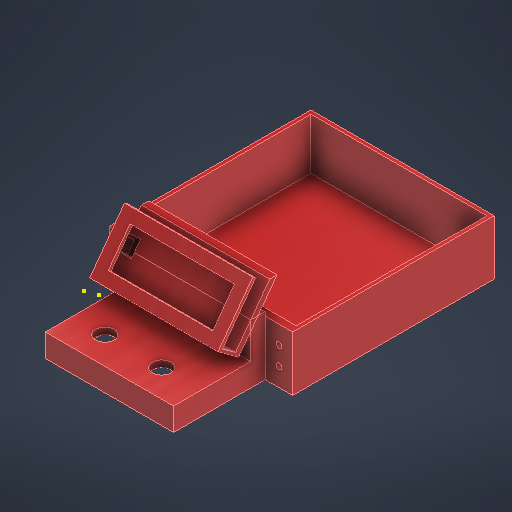
# Autodesk Inventor part: not auger -2.0
Saved by Autodesk Inventor 2026.1 (Build 301233000, 233)
## iProperties
Created: 2025-11-06
Part Number: not auger -2.0
Material: PBT Plastic
Document SubType Name: Modeling
Designer: FrameUser
Density: 1.31 g/cm^3
Appearance: Red
Author: FrameUser
Autodesk Inventor part; units mm, degrees
ref_plane "YZ Plane" through (0, 0, 0) normal (1, 0, 0) x (0, 1, 0)
ref_plane "XZ Plane" through (0, 0, 0) normal (0, 1, 0) x (-1, 0, 0)
ref_plane "XY Plane" through (0, 0, 0) normal (0, 0, 1) x (1, 0, 0)
sketch "Sketch1" plane through (0, 0, 0) normal (0, 1, 0) x (-1, 0, 0)
  line L0 (0, 0) -> (-88.9, 0)
  line L1 (-88.9, 0) -> (-88.9, 63.5)
  line L2 (-88.9, 63.5) -> (0, 63.5)
  line L3 (0, 63.5) -> (0, 0)
  circle A0 centre (-61.675, 44.45) radius 6.5
  circle A1 centre (-22.225, 44.45) radius 6.5
  line L4 (-83.9, 59) -> (-5, 59)
  line L5 (-5, 59) -> (-5, 5)
  line L6 (-5, 5) -> (-83.9, 5)
  line L7 (-83.9, 5) -> (-83.9, 59)
  point P0 (-88.9, 31.75)
  dimension "d0" = 88.9
  dimension "d1" = 63.5
  dimension "d2" = 13
  dimension "d3" = 13
  dimension "d5" = 22.225
  dimension "d8" = 5
  dimension "d9" = 5
  dimension "d10" = 5
  dimension "d11" = 4.5
  dimension "d21" = 19.05
  dimension "d22" = 19.05
  dimension "d78" = 22.225
  constraints: 16 end point, 4 perpendicular, 2 centre point, 2 horizontal, 2 parallel, 1 midpoint
  measures "d0" distance of L0.start L0.end
  measures "d1" distance of L0.end L1.end
  measures "d2" diameter of A0
  measures "d3" diameter of A1
  measures "d5" distance from line of L3 A1.centre
  measures "d8" distance between parallel lines of L7 L1
  measures "d9" distance between parallel lines of L3 L5
  measures "d10" distance between parallel lines of L0 L6
  measures "d11" distance between parallel lines of L2 L4
  measures "d21" distance from line of L2 A0.centre
  measures "d22" distance from line of L2 A1.centre
  measures "d78" distance from line of L7 A0.centre
extrude "Extrusion1" add sketch "Sketch1" along normal blind 15.875 contours L0 L1 L2 L3 | L4 L5 L6 L7
sketch "Sketch2" plane through (0, 0, 0) normal (0, -1, 0) x (1, 0, 0)
  line L0 (83.9, 58.5) -> (5, 58.5)
  line L1 (5, 58.5) -> (5, 5)
  line L2 (5, 5) -> (83.9, 5)
  line L3 (83.9, 5) -> (83.9, 58.5)
  line L4 (0, 63.5) -> (88.9, 63.5) projected
  line L5 (88.9, 63.5) -> (0, 63.5)
  line L6 (0, 63.5) -> (0, 0)
  line L7 (0, 0) -> (88.9, 0)
  line L8 (88.9, 0) -> (88.9, 63.5)
  point P0 (88.9, 31.75)
  point P1 (5, 31.75)
  dimension "d12" = 5
  dimension "d13" = 5
  dimension "d14" = 5
  dimension "d15" = 5
  constraints: 16 end point, 4 parallel, 2 horizontal, 2 midpoint, 2 perpendicular
  measures "d12" distance from line of L3 point (88.9, 31.75)
  measures "d13" distance between parallel lines of L2 L7
  measures "d14" distance from line of L6 point (5, 31.75)
  measures "d15" distance between parallel lines of L4 L0
extrude "Extrusion2" cut sketch "Sketch2" against normal blind 11.35 contours L3 L2 L1 L0
sketch "Sketch3" plane through (0, 15.875, 0) normal (0, 1, 0) x (1, 0, 0)
  line L0 (88.9, -63.5) -> (88.9, 0) projected
  line L1 (0, 0) -> (88.9, 0)
  line L2 (88.9, 0) -> (88.9, -10)
  line L3 (88.9, -10) -> (0, -10)
  line L4 (0, -10) -> (0, 0)
  dimension "d18" = 10
  constraints: 8 end point, 2 parallel, 1 horizontal, 1 perpendicular, 1 point on line
  measures "d18" distance between parallel lines of L3 L1
extrude "Extrusion3" add sketch "Sketch3" along normal blind 25
sketch "Sketch6" plane through (88.9, 0, 0) normal (0, 0, -1) x (-1, 0, 0)
  line L0 (88.9, 0) -> (0, 0)
  line L1 (88.9, 0) -> (88.9, 15.875) projected
  line L2 (0, 0) -> (88.9, 0)
  line L3 (88.9, 0) -> (-38.1, 0)
  line L4 (83.9, 0) -> (5, 0) projected
  line L5 (-19.05, 0) -> (107.95, 0)
  line L6 (107.95, 0) -> (107.95, 38.1)
  line L7 (107.95, 38.1) -> (-19.05, 38.1)
  line L8 (-19.05, 38.1) -> (-19.05, 0)
  circle A0 centre (98.425, 27.2577) radius 2
  circle A1 centre (98.425, 14.4837) radius 2
  line L9 (88.9, 15.875) -> (88.9, 40.875) projected
  line L10 (88.9, 40.875) -> (88.9, 34.3515)
  point P0 (44.45, 0)
  dimension "d32" = 127
  dimension "d33" = 38.1
  dimension "d85" = 4
  dimension "d86" = 4
  dimension "d87" = 9.525
  dimension "d88" = 9.525
  constraints: 16 end point, 3 point on line, 2 centre point, 2 midpoint, 1 collinear, 1 horizontal, 1 perpendicular, 1 vertical
  measures "d32" distance of L5.start L5.end
  measures "d33" distance of L5.end L6.end
  measures "d85" diameter of A0
  measures "d86" diameter of A1
  measures "d87" distance from line of L6 A0.centre
  measures "d88" distance from line of L6 A1.centre
extrude "Extrusion6" add sketch "Sketch6" along normal blind 139.7 contours L0 L3 L8 L7 L9 L1 | L1 L9 L7 L6 L5 | A0 | A1
sketch "Sketch7" plane through (-19.05, 38.1, 0) normal (0, 1, 0) x (1, 0, 0)
  line L0 (124.5, 137.2) -> (2.5, 137.2)
  line L1 (2.5, 137.2) -> (2.5, 5)
  line L2 (2.5, 5) -> (124.5, 5)
  line L3 (124.5, 5) -> (124.5, 137.2)
  line L4 (127, 0) -> (127, 139.7) projected
  line L5 (19.05, 0) -> (0, 0) projected
  line L6 (127, 139.7) -> (0, 139.7)
  line L7 (0, 139.7) -> (0, 0)
  line L8 (0, 0) -> (127, 0)
  line L9 (127, 0) -> (127, 139.7)
  dimension "d36" = 2.5
  dimension "d37" = 2.5
  dimension "d38" = 2.5
  dimension "d39" = 5
  constraints: 16 end point, 4 parallel, 2 horizontal, 2 perpendicular
  measures "d36" distance between parallel lines of L4 L3
  measures "d37" distance between parallel lines of L6 L0
  measures "d38" distance between parallel lines of L7 L1
  measures "d39" distance between parallel lines of L2 L5
extrude "Extrusion7" cut sketch "Sketch7" against normal blind 35.56 contours L3 L2 L1 L0
sketch "Sketch8" plane through (88.9, 0, 63.5) normal (1, 0, 0) x (0, 0, -1)
  line L0 (53.5, 40.875) -> (63.5, 40.875) projected
  line L1 (66.6506, 58.7918) -> (40.3494, 22.9582)
  line L2 (66.6506, 58.7918) -> (71.7306, 58.7918)
  line L3 (71.7306, 58.7918) -> (45.0793, 22.4812)
  line L4 (45.0793, 22.4812) -> (44.4294, 22.9582)
  line L5 (45.0793, 22.4812) -> (30.7458, 33.0017)
  line L6 (30.7458, 33.0017) -> (31.9543, 34.6482)
  line L7 (31.9543, 34.6482) -> (46.2878, 24.1277)
  point P0 (63.5, 0)
  point P1 (58.58, 40.875)
  point P2 (42.9864, 26.5509)
  dimension "d46" = 44.45
  dimension "d47" = 5.08
  dimension "d48" = 17.78
  constraints: 14 end point, 2 perpendicular, 1 horizontal, 1 midpoint, 1 parallel, 1 point on line
  measures "d46" distance of L1.start L1.end
  measures "d47" distance of L1.start L2.end
  measures "d48" distance of L3.end L5.end
extrude "Extrusion8" add sketch "Sketch8" against normal blind 88.9 separate body
sketch "Sketch9" plane through (0, 58.7918, -3.1506) normal (0, 0.5917, 0.8062) x (1, 0, 0)
  point P0 (0, -49.2596)
sketch "Sketch10" plane through (0, 26.5509, 20.5136) normal (0, 0.8062, -0.5917) x (1, 0, 0)
  point P0 (0, 32.2474)
sketch "Sketch11" plane through (0, 26.5509, 20.5136) normal (0, 0.8062, -0.5917) x (1, 0, 0)
  line L0 (88.9, -13.6847) -> (0, -13.6847) projected
  line L1 (0, 4.0953) -> (0, -13.6847) projected
  line L2 (88.9, -13.6847) -> (0, -13.6847)
  line L3 (0, -13.6847) -> (0, -11.1447)
  line L4 (0, -11.1447) -> (88.9, -11.1447)
  line L5 (88.9, -11.1447) -> (88.9, -13.6847)
  point P0 (0, 32.2474)
  dimension "d51" = 2.54
  constraints: 8 end point, 2 parallel, 1 horizontal, 1 perpendicular, 1 point on line
  measures "d51" distance between parallel lines of L0 L4
extrude "Extrusion9" add sketch "Sketch11" along normal blind 44.45 bodies 2
sketch "Sketch12" plane through (0, 33.0017, 32.7542) normal (0, 0.5917, 0.8062) x (1, 0, 0)
  point P0 (0, -7.2238)
sketch "Sketch14" plane through (0, 33.0017, 32.7542) normal (0, 0.5917, 0.8062) x (1, 0, 0)
  line L0 (0, -0.3431) -> (0, -31.9992) projected
  line L1 (0, 0.1776) -> (0, 57.5667)
  line L2 (0, 0.1776) -> (88.9, 0.1776)
  line L3 (88.9, -31.9992) -> (88.9, -0.3431) projected
  line L4 (0, 7.7976) -> (110.0789, 7.7976)
  line L5 (88.9, 46.4924) -> (0, 46.4924) projected
  line L6 (88.9, 46.4924) -> (88.9, 0.1776)
  line L7 (80.645, 0.1776) -> (80.645, 46.4924)
  line L8 (88.9, 45.0417) -> (0, 45.0417) projected
  line L9 (0, 46.4924) -> (0, 0.1776)
  line L10 (8.255, 0.1776) -> (8.255, 51.38)
  line L11 (8.255, 33.1976) -> (80.645, 33.1976)
  line L12 (88.9, 40.8176) -> (0, 40.8176)
  point P0 (0, -7.2238)
  point P1 (80.645, 23.335)
  point P2 (0, 28.8721)
  point P3 (0, 40.8176)
  point P4 (8.255, 7.7976)
  point P5 (80.645, 7.7976)
  dimension "d64" = 7.62
  dimension "d65" = 8.255
  dimension "d66" = 8.255
  dimension "d67" = 25.4
  dimension "d68" = 7.62
  constraints: 18 end point, 9 point on line, 3 perpendicular, 2 collinear, 2 horizontal, 2 midpoint, 2 vertical
  measures "d64" distance between parallel lines of L2 L4
  measures "d65" distance from line of point (80.645, 23.335) L6
  measures "d66" distance from line of L10 point (0, 28.872)
  measures "d67" distance between parallel lines of L4 L11
  measures "d68" distance between parallel lines of L11 L12
extrude "Extrusion10" cut sketch "Sketch14" against normal blind 4.7625 contours L1 L8 L10 L12 | L10 L11 L7 L4 | L10 L8 L7 L12 | L7 L8 L6 L12 bodies 2
sketch "Sketch15" plane through (0, 69.3123, 6.1029) normal (0, -0.8062, 0.5917) x (1, 0, 0)
  line L0 (0, -4.4356) -> (91.0407, -4.4356)
  line L1 (91.0407, -4.4356) -> (91.0407, 6.9043)
  line L2 (91.0407, 6.9043) -> (0, 6.9043)
  line L3 (0, 6.9043) -> (0, -4.4356)
  point P0 (0, -45.9321)
  constraints: 8 end point, 2 parallel, 1 horizontal, 1 perpendicular
extrude "Extrusion11" cut sketch "Sketch15" against normal blind 4.7625 bodies 2
sketch "Sketch16" plane through (105.45, 38.1, -5) normal (0, 0, -1) x (-1, 0, 0)
  circle A0 centre (100.45, -23.5887) radius 5
  point P0 (105.45, -38.1)
  dimension "d73" = 10
  constraints: 1 centre point
  measures "d73" diameter of A0
extrude "Extrusion12" cut sketch "Sketch16" against normal blind 19.05 bodies 1
sketch "Sketch18" plane through (0, 58.7918, -3.1506) normal (0, 0.5917, 0.8062) x (1, 0, 0)
  line L0 (0, -39.9934) -> (0, 0) projected
  line L1 (0, -39.9934) -> (0, -25.4934)
  line L2 (0, -25.4934) -> (0, -14.9934)
  line L3 (0, -14.9934) -> (8, -14.9934)
  line L4 (8, -14.9934) -> (8, -25.4934)
  line L5 (8, -25.4934) -> (0, -25.4934)
  point P0 (0, -49.2596)
  dimension "d80" = 14.5
  dimension "d81" = 10.5
  dimension "d82" = 8
  constraints: 10 end point, 2 perpendicular, 2 point on line, 1 vertical
  measures "d80" distance of L0.start L1.end
  measures "d81" distance of L1.end L2.end
  measures "d82" distance of L2.end L3.end
extrude "Extrusion14" cut sketch "Sketch18" against normal blind 7 bodies 2 1
sketch "Sketch19" plane through (88.9, 0, 0) normal (0, 0, 1) x (1, 0, 0)
  circle A0 centre (-98.425, 25.4) radius 2
  circle A1 centre (-98.425, 12.7) radius 2
  line L0 (-107.95, 0) -> (-107.95, 38.1) projected
  circle A2 centre (9.525, 25.4) radius 2
  circle A3 centre (9.525, 12.7) radius 2
  line L1 (19.05, 38.1) -> (19.05, 0) projected
  line L2 (-107.95, 38.1) -> (19.05, 38.1) projected
  point P0 (-88.9, 0)
  dimension "d89" = 4
  dimension "d90" = 4
  dimension "d91" = 9.525
  dimension "d92" = 9.525
  dimension "d93" = 4
  dimension "d94" = 4
  dimension "d95" = 9.525
  dimension "d96" = 9.525
  dimension "d97" = 12.7
  dimension "d98" = 12.7
  dimension "d99" = 12.7
  dimension "d100" = 12.7
  constraints: 4 centre point
  measures "d89" diameter of A0
  measures "d90" diameter of A1
  measures "d91" distance from line of L0 A0.centre
  measures "d92" distance from line of L0 A1.centre
  measures "d93" diameter of A2
  measures "d94" diameter of A3
  measures "d95" distance from line of L1 A2.centre
  measures "d96" distance from line of L1 A3.centre
  measures "d97" distance from line of L2 A2.centre
  measures "d98" distance of A2.centre A3.centre
  measures "d99" distance from line of L2 A0.centre
  measures "d100" distance of A0.centre A1.centre
extrude "Extrusion15" cut sketch "Sketch19" against normal blind 19.05 bodies 1
sketch "Sketch20" plane through (5, 0, 5) normal (0, 0, 1) x (1, 0, 0)
  arc A0 (46.0235, 3.0327) -> (33.3235, 3.0327) centre (39.6735, 3.0327) ccw
  line L0 (46.0235, 3.0327) -> (46.0235, 1.34)
  line L1 (46.0235, 1.34) -> (33.3235, 1.34)
  line L2 (33.3235, 1.34) -> (33.3235, 3.0327)
  point P0 (-5, 0)
  dimension "d106" = 12.7
  constraints: 6 end point, 2 perpendicular, 2 point on circle, 1 centre point, 1 tangent, 1 vertical
  measures "d106" distance of L2.end L0.start
extrude "Extrusion16" cut sketch "Sketch20" against normal blind 20.6375 bodies 1
body "Solid1"
body "Solid2"
